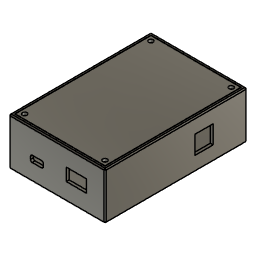
Enclosure (Autodesk Fusion 360 design; units mm, degrees)
Autodesk Fusion 360 part; units mm, degrees
sketch "Sketch1" plane through (0, 0, 0) normal (0, 0, 1) x (1, 0, 0)
  line L0 (28, 58.0885) -> (-35, 58.0885)
  line L1 (-35, 58.0885) -> (-35, -36.9115)
  line L2 (-35, -36.9115) -> (28, -36.9115)
  line L3 (28, -36.9115) -> (28, 58.0885)
  line L4 (28, 58.0885) -> (-35, -36.9115) construction
  line L5 (-35, 58.0885) -> (28, -36.9115) construction
  line L6 (-37, -38.9115) -> (30, -38.9115)
  line L7 (30, -38.9115) -> (30, 60.0885)
  line L8 (30, 60.0885) -> (-37, 60.0885)
  line L9 (-37, 60.0885) -> (-37, -38.9115)
  point P0 (-3.5, 10.5885)
  dimension "d1" = 63
  dimension "d2" = 95
  dimension "d3" = 2
  constraint horizontal L0
  constraint perpendicular L0 L1
  constraint parallel L0 L2
  constraint parallel L1 L3
  constraint coincident L4 P0
  constraint coincident L5 P0
  measures "d1" distance of L1.end L2.end
  measures "d2" distance of L0.end L1.end
extrude "Extrude1" add sketch "Sketch1" against normal blind 2 contours L0 L1 L2 L3 | L6 L7 L8 L9 makes body 1
extrude "Extrude2" add sketch "Sketch1" along normal blind 31 bodies 1
sketch "Sketch2" plane through (30, 0, 0) normal (1, 0, 0) x (0, 1, 0)
  line L0 (-38.9115, 31) -> (-38.9115, -2)
  line L1 (-38.9115, -2) -> (60.0885, -2)
  line L2 (60.0885, -2) -> (60.0885, 31)
  line L3 (60.0885, 31) -> (-38.9115, 31)
  line L4 (60.0885, 14.5) -> (30.0885, 14.5)
  line L5 (23.7385, 20.875) -> (36.4385, 20.875)
  line L6 (36.4385, 20.875) -> (36.4385, 8.125)
  line L7 (36.4385, 8.125) -> (23.7385, 8.125)
  line L8 (23.7385, 8.125) -> (23.7385, 20.875)
  line L9 (23.7385, 20.875) -> (36.4385, 8.125) construction
  line L10 (36.4385, 20.875) -> (23.7385, 8.125) construction
  point P0 (30.0885, 14.5)
  dimension "d8" = 30
  dimension "d9" = 12.7
  dimension "d10" = 12.75
  constraint midpoint L2 L4.start
  constraint perpendicular L2 L4
  constraint horizontal L5
  constraint perpendicular L5 L6
  constraint parallel L5 L7
  constraint parallel L6 L8
  constraint coincident L9 P0
  constraint coincident L10 P0
  constraint coincident P0 L4.end
  measures "d8" distance of L4.start P0
  measures "d9" distance of L6.end L7.end
  measures "d10" distance of L5.end L6.end
extrude "Extrude3" cut sketch "Sketch2" against normal blind 76 contours L5 L6 L7 L8 bodies 1
sketch "Sketch3" plane through (0, -38.9115, 0) normal (0, -1, 0) x (1, 0, 0)
  line L0 (-37, 31) -> (-37, -2)
  line L1 (-37, -2) -> (30, -2)
  line L2 (30, -2) -> (30, 31)
  line L3 (30, 31) -> (-37, 31)
  line L4 (-37, -2) -> (-22, -2)
  line L5 (-22, -2) -> (-22, 9.8)
  line L6 (-22, 9.8) -> (-37, 9.8)
  line L7 (-37, 9.8) -> (-37, -2)
  line L8 (-22, 9.8) -> (-13, 9.8)
  line L9 (-13, 9.8) -> (-13, 14.2)
  line L10 (-13, 14.2) -> (-22, 14.2)
  line L11 (-22, 14.2) -> (-22, 9.8)
  line L12 (30, 14.5) -> (10, 14.5)
  line L13 (17, 10.15) -> (3, 10.15)
  line L14 (3, 10.15) -> (3, 18.85)
  line L15 (3, 18.85) -> (17, 18.85)
  line L16 (17, 18.85) -> (17, 10.15)
  line L17 (17, 10.15) -> (3, 18.85) construction
  line L18 (3, 10.15) -> (17, 18.85) construction
  point P0 (10, 14.5)
  dimension "d13" = 15
  dimension "d14" = 11.8
  dimension "d15" = 9
  dimension "d16" = 4.4
  dimension "d17" = 14
  dimension "d18" = 8.7
  dimension "d19" = 20
  constraint horizontal L4
  constraint vertical L5
  constraint horizontal L6
  constraint vertical L7
  constraint coincident L0.end L1.start
  constraint horizontal L8
  constraint vertical L9
  constraint horizontal L10
  constraint vertical L11
  constraint midpoint L2 L12.start
  constraint perpendicular L2 L12
  constraint horizontal L13
  constraint perpendicular L13 L14
  constraint parallel L13 L15
  constraint parallel L14 L16
  constraint coincident L17 P0
  constraint coincident L18 P0
  constraint coincident P0 L12.end
  measures "d13" distance of L0.end L4.end
  measures "d14" distance of L0.end L6.end
  measures "d15" distance of L9.end L10.end
  measures "d16" distance of L8.end L9.end
  measures "d17" distance of L14.end L15.end
  measures "d18" distance of L13.start L15.end
  measures "d19" distance of L12.start P0
extrude "Extrude4" cut sketch "Sketch3" against normal blind 3 contours L8 L9 L10 L11 | L13 L14 L15 L16 bodies 1
sketch "Sketch4" plane through (0, 60.0885, 0) normal (0, 1, 0) x (-1, 0, 0)
  line L0 (-30, 31) -> (-30, -2)
  line L1 (-30, -2) -> (37, -2)
  line L2 (37, -2) -> (37, 31)
  line L3 (37, 31) -> (-30, 31)
  line L4 (3.5, -2) -> (3.5, 31)
  line L5 (3.5, 14.5) -> (-10, 14.5)
  circle A0 centre (-10, 14.5) radius 2.1
  line L6 (3.5, 14.5) -> (17, 14.5)
  circle A1 centre (17, 14.5) radius 2.1
  dimension "d22" = 13.5
  dimension "d23" = 4.2
  constraint midpoint L1 L4.start
  constraint midpoint L3 L4.end
  constraint midpoint L4 L5.start
  constraint perpendicular L4 L5
  constraint coincident L5.end A0.centre
  constraint symmetric L4 L5.start L6.start
  constraint symmetric L4 L5.end L6.end
  constraint symmetric L4 A0 A1
  measures "d22" distance of L5.start L5.end
  measures "d23" diameter of A0
extrude "Extrude5" cut sketch "Sketch4" against normal blind 3 contours A0 | A1 bodies 1
chamfer "Chamfer1" distance 0.8 angle 45 12 edges at (30, 10.5885, 31) (-3.5, -38.9115, 31) (-37, 10.5885, 31) (-3.5, 60.0885, 31) (30, -38.9115, 14.5) (-37, -38.9115, 14.5) (-3.5, -38.9115, -2) (30, 10.5885, -2) (30, 60.0885, 14.5) (-3.5, 60.0885, -2) (-37, 60.0885, 14.5) (-37, 10.5885, -2) on bodies 1
sketch "Sketch6" plane through (0, 0, 31) normal (0, 0, 1) x (-1, 0, 0)
  line L0 (-28, -58.0885) -> (-28, 36.9115)
  line L1 (-28, 36.9115) -> (35, 36.9115)
  line L2 (35, 36.9115) -> (35, -58.0885)
  line L3 (35, -58.0885) -> (-28, -58.0885)
  line L4 (-29.2, -59.2885) -> (36.2, -59.2885)
  line L5 (36.2, -59.2885) -> (36.2, 38.1115)
  line L6 (36.2, 38.1115) -> (-29.2, 38.1115)
  line L7 (-29.2, 38.1115) -> (-29.2, -59.2885)
  line L8 (35, -58.0885) -> (28, -58.0885)
  line L9 (28, -58.0885) -> (28, -51.0885)
  line L10 (28, -51.0885) -> (35, -51.0885)
  line L11 (35, -51.0885) -> (35, -58.0885)
  line L12 (-28, 36.9115) -> (-21, 36.9115)
  line L13 (-21, 36.9115) -> (-21, 29.9115)
  line L14 (-21, 29.9115) -> (-28, 29.9115)
  line L15 (-28, 29.9115) -> (-28, 36.9115)
  line L16 (35, 36.9115) -> (28, 36.9115)
  line L17 (28, 36.9115) -> (28, 29.9115)
  line L18 (28, 29.9115) -> (35, 29.9115)
  line L19 (35, 29.9115) -> (35, 36.9115)
  line L20 (-28, -58.0885) -> (-21, -58.0885)
  line L21 (-21, -58.0885) -> (-21, -51.0885)
  line L22 (-21, -51.0885) -> (-28, -51.0885)
  line L23 (-28, -51.0885) -> (-28, -58.0885)
  line L24 (28, 29.9115) -> (31.5, 29.9115)
  line L25 (31.5, 29.9115) -> (31.5, 33.4115)
  line L26 (31.5, 33.4115) -> (28, 33.4115)
  line L27 (28, 33.4115) -> (28, 29.9115)
  line L28 (-21, 29.9115) -> (-24.4742, 29.9115)
  line L29 (-24.4742, 29.9115) -> (-24.4742, 33.4115)
  line L30 (-24.4742, 33.4115) -> (-21, 33.4115)
  line L31 (-21, 33.4115) -> (-21, 29.9115)
  line L32 (-21, -51.0885) -> (-24.5, -51.0885)
  line L33 (-24.5, -51.0885) -> (-24.5, -54.5885)
  line L34 (-24.5, -54.5885) -> (-21, -54.5885)
  line L35 (-21, -54.5885) -> (-21, -51.0885)
  line L36 (28, -51.0885) -> (31.5, -51.0885)
  line L37 (31.5, -51.0885) -> (31.5, -54.5885)
  line L38 (31.5, -54.5885) -> (28, -54.5885)
  line L39 (28, -54.5885) -> (28, -51.0885)
  circle A0 centre (31.5, -54.5885) radius 2.2
  circle A1 centre (-24.5, -54.5885) radius 2.2
  circle A2 centre (-24.4742, 33.4115) radius 2.2
  circle A3 centre (31.5, 33.4115) radius 2.2
  circle A4 centre (31.5, 33.4115) radius 1.6
  circle A5 centre (-24.4742, 33.4115) radius 1.6
  circle A6 centre (31.5, -54.5885) radius 1.6
  circle A7 centre (-24.5, -54.5885) radius 1.6
  dimension "d30" = 7
  dimension "d31" = 7
  dimension "d32" = 7
  dimension "d33" = 7
  dimension "d34" = 7
  dimension "d35" = 7
  dimension "d36" = 7
  dimension "d37" = 7
  dimension "d40" = 4.4
  dimension "d41" = 4.4
  dimension "d42" = 4.4
  dimension "d43" = 4.4
  dimension "d51" = 3.2
  dimension "d52" = 3.2
  dimension "d53" = 3.2
  dimension "d54" = 3.2
  constraint horizontal L8
  constraint vertical L9
  constraint horizontal L10
  constraint vertical L11
  constraint coincident L2.end L3.start
  constraint horizontal L12
  constraint vertical L13
  constraint horizontal L14
  constraint vertical L15
  constraint coincident L0.end L1.start
  constraint horizontal L16
  constraint vertical L17
  constraint horizontal L18
  constraint vertical L19
  constraint coincident L1.end L2.start
  constraint horizontal L20
  constraint vertical L21
  constraint horizontal L22
  constraint vertical L23
  constraint coincident L0.start L3.end
  constraint horizontal L24
  constraint vertical L25
  constraint horizontal L26
  constraint vertical L27
  constraint horizontal L28
  constraint vertical L29
  constraint horizontal L30
  constraint vertical L31
  constraint horizontal L32
  constraint vertical L33
  constraint horizontal L34
  constraint vertical L35
  constraint horizontal L36
  constraint vertical L37
  constraint horizontal L38
  constraint vertical L39
  constraint coincident L37.end L38.start
  constraint coincident L33.end L34.start
  constraint coincident L29.end L30.start
  constraint coincident L25.end L26.start
  constraint concentric A2 A5
  constraint concentric A0 A6
  constraint concentric A1 A7
  measures "d30" distance of L2.end L8.end
  measures "d31" distance of L2.end L10.end
  measures "d32" distance of L0.end L12.end
  measures "d33" distance of L0.end L14.end
  measures "d34" distance of L1.end L16.end
  measures "d35" distance of L1.end L18.end
  measures "d36" distance of L0.start L20.end
  measures "d37" distance of L0.start L22.end
  measures "d40" diameter of A0
  measures "d41" diameter of A1
  measures "d42" diameter of A2
  measures "d43" diameter of A3
  measures "d51" diameter of A4
  measures "d52" diameter of A5
  measures "d53" diameter of A6
  measures "d54" diameter of A7
extrude "Extrude7" add sketch "Sketch6" against normal blind 18 contours L0 L3 L20 L21 L22 L23 L33 L34 A1 | L0 L1 L12 L13 L14 L15 L29 L30 A2 | L21 L22 L32 L33 L34 L35 A1 | L2 L3 L8 L9 L10 L11 L37 L38 A0 | L13 L14 L28 L29 L30 L31 A2 | L33 L34 A1 A7 | L33 L34 A1 A7 | L9 L10 L36 L37 L38 L39 A0 | L29 L30 A2 A5 | L29 L30 A2 A5 | L33 L34 A7 | L33 L34 A7 | L37 L38 A0 A6 | L37 L38 A0 A6 | L1 L2 L16 L17 L18 L19 L25 L26 A3 | L29 L30 A5 | L29 L30 A5 | L37 L38 A6 | L37 L38 A6 | L17 L18 L24 L25 L26 L27 A3 | L25 L26 A3 A4 | L25 L26 A3 A4 | L25 L26 A4 | L25 L26 A4 bodies 1
extrude "Extrude8" cut sketch "Sketch6" against normal blind 2.1 contours L0 L3 L20 L21 L22 L23 L33 L34 A1 | L0 L1 L12 L13 L14 L15 L29 L30 A2 | L21 L22 L32 L33 L34 L35 A1 | L2 L3 L8 L9 L10 L11 L37 L38 A0 | L13 L14 L28 L29 L30 L31 A2 | L9 L10 L36 L37 L38 L39 A0 | L1 L2 L16 L17 L18 L19 L25 L26 A3 | L17 L18 L24 L25 L26 L27 A3 bodies 1
extrude "Extrude9" cut sketch "Sketch6" against normal blind 10.2 contours L33 L34 A1 A7 | L33 L34 A1 A7 | L29 L30 A2 A5 | L29 L30 A2 A5 | L33 L34 A7 | L33 L34 A7 | L37 L38 A0 A6 | L37 L38 A0 A6 | L29 L30 A5 | L29 L30 A5 | L37 L38 A6 | L37 L38 A6 | L25 L26 A3 A4 | L25 L26 A3 A4 | L25 L26 A4 | L25 L26 A4 bodies 1
chamfer "Chamfer2" distance 7 angle 45 8 edges at (-28, 54.5885, 13) (-31.5, 51.0885, 13) (24.5, 51.0885, 13) (21, 54.5885, 13) (-31.5, -29.9115, 13) (24.5, -29.9115, 13) (-28, -33.4115, 13) (21, -33.4115, 13) on bodies 1
sketch "Sketch5" plane through (0, 0, 31) normal (0, 0, 1) x (-1, 0, 0)
  line L0 (-28, -58.0885) -> (-28, 36.9115)
  line L1 (-28, 36.9115) -> (35, 36.9115)
  line L2 (35, 36.9115) -> (35, -58.0885)
  line L3 (35, -58.0885) -> (-28, -58.0885)
  line L4 (-27.85, 36.7615) -> (34.85, 36.7615)
  line L5 (34.85, 36.7615) -> (34.85, -57.9385)
  line L6 (34.85, -57.9385) -> (-27.85, -57.9385)
  line L7 (-27.85, -57.9385) -> (-27.85, 36.7615)
  line L8 (-29.2, -59.2885) -> (36.2, -59.2885)
  line L9 (36.2, -59.2885) -> (36.2, 38.1115)
  line L10 (36.2, 38.1115) -> (-29.2, 38.1115)
  line L11 (-29.2, 38.1115) -> (-29.2, -59.2885)
  dimension "d26" = 0.15
extrude "Extrude6" add sketch "Sketch5" against normal blind 2 separate body contours L4 L5 L6 L7 makes body 2
extrude "Extrude11" cut sketch "Sketch6" against normal blind 2 contours L33 L34 A7 | L33 L34 A7 | L29 L30 A5 | L29 L30 A5 | L37 L38 A6 | L37 L38 A6 | L25 L26 A4 | L25 L26 A4 bodies 2
sketch "Sketch7" plane through (0, -36.9115, 0) normal (0, 1, 0) x (-1, 0, 0)
  line L0 (-28, 13) -> (-28, 0)
  line L1 (-28, 0) -> (35, 0)
  line L2 (35, 0) -> (35, 13)
  line L3 (35, 13) -> (28, 20)
  line L4 (28, 20) -> (28, 28.9)
  line L5 (28, 28.9) -> (35, 28.9)
  line L6 (35, 28.9) -> (35, 31)
  line L7 (35, 31) -> (-28, 31)
  line L8 (-28, 31) -> (-28, 28.9)
  line L9 (-28, 28.9) -> (-21, 28.9)
  line L10 (-21, 28.9) -> (-21, 20)
  line L11 (-21, 20) -> (-28, 13)
  line L12 (-3, 18.85) -> (-3, 10.15)
  line L13 (-3, 10.15) -> (-17, 10.15)
  line L14 (-17, 10.15) -> (-17, 18.85)
  line L15 (-17, 18.85) -> (-3, 18.85)
  line L16 (22, 9.8) -> (13, 9.8)
  line L17 (13, 9.8) -> (13, 14.2)
  line L18 (13, 14.2) -> (22, 14.2)
  line L19 (22, 14.2) -> (22, 9.8)
  line L20 (13, 9.8) -> (7, 9.8)
  line L21 (7, 9.8) -> (7, 6.3)
  line L22 (7, 6.3) -> (13, 6.3)
  line L23 (13, 6.3) -> (13, 9.8)
  line L24 (13, 9.8) -> (28, 9.8)
  line L25 (28, 9.8) -> (28, 6.5)
  line L26 (28, 6.5) -> (13, 6.5)
  line L27 (13, 6.5) -> (13, 9.8)
  dimension "d57" = 6
  dimension "d58" = 3.5
  dimension "d59" = 15
  constraint horizontal L20
  constraint vertical L21
  constraint horizontal L22
  constraint vertical L23
  constraint coincident L16.end L17.start
  constraint horizontal L24
  constraint vertical L25
  constraint horizontal L26
  constraint vertical L27
  measures "d57" distance of L16.end L20.end
  measures "d58" distance of L16.end L22.end
  measures "d59" distance of L16.end L24.end
extrude "Extrude12" add sketch "Sketch7" along normal blind 30 separate body contours L16 L23 L24 L25 L26 L27 | L20 L21 L22 L23 L27 makes body 3
fillet "Fillet1" radius 1.2 4 edges at (-13, -37.9115, 14.2) (-13, -37.9115, 9.8) (-22, -37.9115, 9.8) (-22, -37.9115, 14.2) on bodies 1
equation "d1 = 70 mm - 7 mm"
equation "d2 = 115 mm - 20 mm"
equation "d22 = ( 27 / 2 ) * 1 mm"
equation "d59 = 9 mm + 6 mm"
